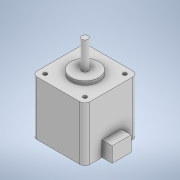
# Autodesk Inventor part: stepperMotor
Saved by Autodesk Inventor 2021 (Build 250183000, 183)
## iProperties
Created: 2021-03-14
Part Number: stepperMotor
Material: Generic
Document SubType Name: Modeling
Designer: awitc
Density: 1 g/cm^3
Appearance: Default
Author: awitc
Autodesk Inventor part; units mm, degrees
ref_plane "YZ Plane" through (0, 0, 0) normal (1, 0, 0) x (0, 1, 0)
ref_plane "XZ Plane" through (0, 0, 0) normal (0, 1, 0) x (-1, 0, 0)
ref_plane "XY Plane" through (0, 0, 0) normal (0, 0, 1) x (1, 0, 0)
sketch "Sketch1" plane through (0, 0, 0) normal (0, 1, 0) x (-1, 0, 0)
  line L0 (0, 0) -> (42, 0)
  line L1 (42, 0) -> (42, -42)
  line L2 (42, -42) -> (0, -42)
  line L3 (0, -42) -> (0, 0)
  line L4 (42, -21) -> (42, -5.25)
  line L5 (21, -5.25) -> (36.75, -5.25)
  line L6 (36.75, -5.25) -> (5.25, -5.25)
  line L7 (5.25, -5.25) -> (5.25, -36.75)
  line L8 (5.25, -36.75) -> (36.75, -36.75)
  line L9 (36.75, -36.75) -> (36.75, -5.25)
  circle A0 centre (36.75, -5.25) radius 1.5
  circle A1 centre (36.75, -36.75) radius 1.5
  circle A2 centre (5.25, -36.75) radius 1.5
  circle A3 centre (5.25, -5.25) radius 1.5
  dimension "d6" = 3
  dimension "d7" = 3
  dimension "d8" = 3
  dimension "d9" = 3
  constraints: 20 end point, 4 centre point, 4 coincident, 4 parallel, 2 horizontal, 2 perpendicular, 1 midpoint, 1 point on line
  measures "d6" diameter of A0
  measures "d7" diameter of A1
  measures "d8" diameter of A2
  measures "d9" diameter of A3
extrude "Extrusion1" add sketch "Sketch1" along normal blind 43 contours L0 L1 L2 L3 | L5 A0 L9 A1 L8 A2 L7 A3 L6
sketch "Sketch2" plane through (0, 43, 0) normal (0, 1, 0) x (1, 0, 0)
  circle A0 centre (-21, 21) radius 11
  circle A1 centre (-21, 21) radius 2.5
  point P0 (0, 0)
  dimension "d12" = 22
  dimension "d15" = 5
  constraints: 2 centre point, 1 coincident
  measures "d12" diameter of A0
  measures "d15" diameter of A1
extrude "Extrusion2" add sketch "Sketch2" along normal blind 3 contours A0 | A1
extrude "Extrusion3" add sketch "Sketch2" along normal blind 25 contours A1
sketch "Sketch3" plane through (0, 0, 0) normal (1, 0, 0) x (0, 0, -1)
  line L0 (42, 0) -> (0, 0) projected
  line L1 (21, 0) -> (28.5, 0)
  line L2 (28.5, 0) -> (13.5, 0)
  line L3 (13.5, 0) -> (13.5, 12)
  line L4 (13.5, 12) -> (28.5, 12)
  line L5 (28.5, 12) -> (28.5, 0)
  dimension "d18" = 7.5
  dimension "d19" = 15
  dimension "d20" = 12
  constraints: 10 end point, 3 perpendicular, 2 point on line, 1 midpoint
  measures "d18" distance of L1.start L1.end
  measures "d19" distance of L1.end L2.end
  measures "d20" distance of L2.end L3.end
extrude "Extrusion4" add sketch "Sketch3" along normal blind 8
fillet "Fillet1" radius 4 4 edges at (0, 21.5, 0) (0, 21.5, -42) (-42, 21.5, 0) (-42, 21.5, -42)
body "Solid1"
